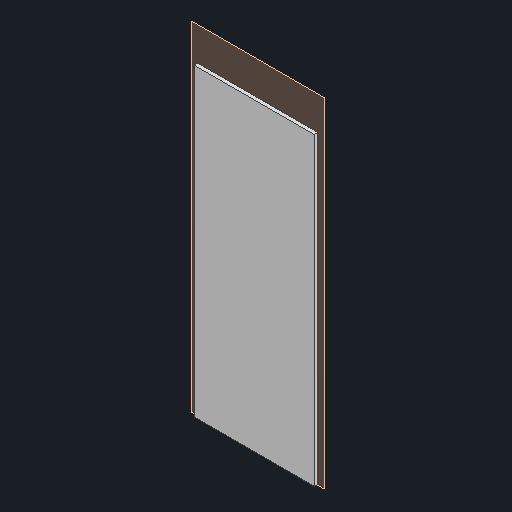
# Autodesk Inventor part: right_metal_gear_bracker
Saved by Autodesk Inventor 2023 (Build 270158000, 158)
## iProperties
Created: 2024-04-23
Part Number: right_metal_gear_bracker
Material: Generic
Document SubType Name: Modeling
Designer: szymo
Density: 1 g/cm^3
Appearance: Default
Author: szymo
Autodesk Inventor part; units mm, degrees
ref_plane "YZ Plane" through (0, 0, 0) normal (1, 0, 0) x (0, 1, 0)
ref_plane "XZ Plane" through (0, 0, 0) normal (0, 1, 0) x (-1, 0, 0)
ref_plane "XY Plane" through (0, 0, 0) normal (0, 0, 1) x (1, 0, 0)
ref_plane "Work Plane1" through (3, 4, -1) normal (0, 0, 1) x (0, -1, 0)
sketch "Sketch1" plane through (3, 4, -1) normal (0, 0, 1) x (0, -1, 0)
  line L0 (89.75, 33.5) -> (5, 33.5) projected
  line L1 (5, 0) -> (5, 33.5) projected
  line L2 (5, 0) -> (89.75, 0) projected
  line L3 (89.75, 0) -> (89.75, 33.5) projected
  line L4 (5, 0) -> (60, 0) projected
  line L5 (5, -3) -> (5, 0) projected
  line L6 (4, -3) -> (60, -3) projected
  line L7 (183, 4.5) -> (137.8889, 33.5) projected
  line L8 (137.8889, 33.5) -> (60, 33.5) projected
  line L9 (60, 33.5) -> (60, 3.25) projected
  line L10 (60, -3) -> (60, 0) projected
  line L11 (183, 0) -> (183, 4.5) projected
  arc A0 (63.25, 0) -> (60, 3.25) centre (63.25, 3.25) ccw projected
  line L12 (88.5, 0) -> (183, 0) projected
  line L13 (63.25, 0) -> (88.5, 0) projected
  circle A1 centre (88.5, 3.25) radius 3.25 projected
  point P0 (52, 0)
  point P1 (64.076, 0)
  point P2 (87.674, 0)
  constraints: 1 vertical alignment
extrude "Extrusion1" add sketch "Sketch1" along normal blind 1 contours L3 A1 L2 A0 L9 L0 | L9 A0 L2 L1 L0 | L3 A1 | L3 L2 A1 picked at (88.2632, 3.0814)
body "Solid1"
